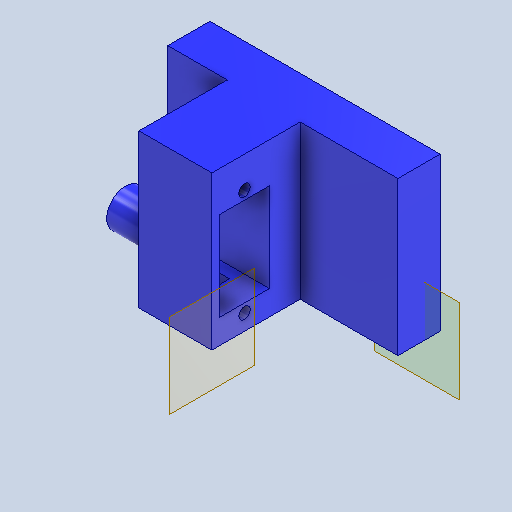
# Autodesk Inventor part: joint5_cover
Saved by Autodesk Inventor 2022 (Build 260153000, 153)
## iProperties
Created: 2024-10-12
Part Number: joint5_cover
Material: 一般
Document SubType Name: Modeling
Designer: acbaf
Density: 1 g/cm^3
Appearance: 青 - 壁塗料 - 光沢
Author: acbaf
Autodesk Inventor part; units mm, degrees
ref_plane "YZ Plane" through (0, 0, 0) normal (1, 0, 0) x (0, 1, 0)
sketch "スケッチ12" plane through (0, 0, 0) normal (1, 0, 0) x (0, 1, 0)
  line L0 (0, 0) -> (-40, 0)
  line L1 (-40, 0) -> (-40, -30)
  line L2 (-40, -30) -> (0, -30)
  line L3 (0, -30) -> (0, 0)
  dimension "d86" = 40
  dimension "d87" = 30
  constraints: 8 end point, 2 parallel, 1 horizontal, 1 perpendicular
  measures "d86" distance of L2.end L1.end
  measures "d87" distance of L1.end L0.end
extrude "押し出し15" add sketch "スケッチ12" along normal blind 60
sketch "スケッチ13" plane through (60, 0, 0) normal (1, 0, 0) x (0, 0, -1)
  line L0 (0, 0) -> (0, -2)
  line L1 (2, -10.4) -> (15, -10.4)
  line L2 (15, -10.4) -> (15, -33.6)
  line L3 (15, -33.6) -> (2, -33.6)
  line L4 (2, -33.6) -> (2, -10.4)
  line L5 (30, 0) -> (0, 0) projected
  line L6 (30, -40) -> (30, 0) projected
  line L7 (0, 0) -> (0, -40) projected
  line L8 (0, -40) -> (30, -40) projected
  line L9 (30, -40) -> (30, 0) projected
  line L10 (30, 0) -> (0, 0) projected
  line L11 (0, 0) -> (0, -40) projected
  line L12 (0, -40) -> (30, -40) projected
  line L13 (23, -40) -> (23, 0)
  point P0 (-10, 3.6606)
  point P1 (23, 0)
  point P2 (8.5, -27.6)
  dimension "d94" = 23.2
  dimension "d95" = 10.4
  dimension "d99" = 13
  dimension "d130" = 8
  dimension "d137" = 6
  dimension "d138" = 6.5
  dimension "d145" = 15
  dimension "d146" = 2
  constraints: 12 end point, 2 parallel, 2 perpendicular, 2 point on line, 1 horizontal
  measures "d94" distance of L1.end L2.end
  measures "d95" distance between parallel lines of L1 L5
  measures "d99" distance of L1.start L1.end
  measures "d130" distance between parallel lines of L13 L2
  measures "d137" distance from line of L3 point (8.5, -27.6)
  measures "d138" distance from line of point (8.5, -27.6) L4
  measures "d145" distance between parallel lines of L2 L6
  measures "d146" distance between parallel lines of L7 L4
extrude "押し出し16" cut sketch "スケッチ13" against normal blind 16.4 contours L1 L2 L3 L4
sketch "スケッチ14" plane through (0, -40, -30) normal (0, 0, -1) x (-1, 0, 0)
  line L0 (0, 0) -> (0, 40) projected
  line L1 (0, 40) -> (-60, 40) projected
  line L2 (-60, 0) -> (-60, 40) projected
  line L3 (0, 0) -> (-60, 0) projected
  circle A0 centre (-30, 20) radius 2.7
  circle A1 centre (-30, 20) radius 4.75
  line L4 (-30, 20) -> (-54, 20)
  line L5 (-30, 20) -> (-6, 20)
  circle A2 centre (-30, 20) radius 6.5
  circle A3 centre (-6, 20) radius 4
  line L6 (-30, 13.5) -> (-30, 26.5)
  circle A4 centre (-54, 20) radius 4
  line L7 (-29.3229, 13.5354) -> (-5.5833, 16.0218)
  line L8 (-5.5833, 23.9782) -> (-29.3229, 26.4646)
  line L9 (-30.6771, 26.4646) -> (-54.4167, 23.9782)
  line L10 (-30.6771, 13.5354) -> (-54.4167, 16.0218)
  circle A5 centre (-54, 20) radius 0.5
  circle A6 centre (-50, 20) radius 0.5
  circle A7 centre (-46, 20) radius 0.5
  circle A8 centre (-42, 20) radius 0.5
  circle A9 centre (-38, 20) radius 0.5
  circle A10 centre (-6, 20) radius 0.5
  circle A11 centre (-10, 20) radius 0.5
  circle A12 centre (-14, 20) radius 0.5
  circle A13 centre (-18, 20) radius 0.5
  circle A14 centre (-22, 20) radius 0.5
  line L11 (44.5, 22.6) -> (44.5, 22.6)
  line L12 (-15.5, 0) -> (-15.5, 0)
  line L13 (-46.2012, 14.0596) -> (-13.7988, 25.9404)
  line L14 (44.5, 0) -> (44.5, 0)
  line L15 (-15.5, 22.6) -> (-15.5, 22.6)
  line L16 (44.5, 22.6) -> (44.5, 22.6)
  line L17 (44.5, 22.6) -> (-15.5, 0)
  line L18 (44.5, 22.6) -> (-15.5, 22.6)
  line L19 (-15.5, 22.6) -> (44.5, 0)
  point P0 (16, 11.6)
  point P1 (-30, 20)
  point P2 (14.5, 11.3)
  dimension "d170" = 5.4
  dimension "d171" = 9.5
  dimension "d172" = 24
  dimension "d173" = 24
  dimension "d174" = 13
  dimension "d175" = 8
  dimension "d176" = 0
  dimension "d177" = 0
  dimension "d178" = 1
  dimension "d179" = 1
  dimension "d180" = 4
  dimension "d181" = 1
  dimension "d182" = 1
  dimension "d183" = 1
  dimension "d184" = 4
  dimension "d185" = 4
  dimension "d186" = 4
  dimension "d187" = 30
  dimension "d188" = 20
  constraints: 32 end point, 15 centre point, 10 point on circle, 8 tangent, 6 coincident, 6 symmetric about line, 5 midpoint, 3 point on line, 6 other
  measures "d170" diameter of A0
  measures "d171" diameter of A1
  measures "d172" distance of L4.start L4.end
  measures "d173" distance of L4.start L5.end
  measures "d174" diameter of A2
  measures "d175" diameter of A3
  measures "d176" distance from line of L4 A4.centre
  measures "d177" distance from line of L6 A0.centre
  measures "d178" diameter of A5
  measures "d179" diameter of A6
  measures "d180" distance of L4.end A6.centre
  measures "d181" diameter of A7
  measures "d182" diameter of A8
  measures "d183" diameter of A9
  measures "d184" distance of A6.centre A7.centre
  measures "d185" distance of A7.centre A8.centre
  measures "d186" distance of A9.centre A8.centre
  measures "d187" distance from line of L2 point (-30, 20)
  measures "d188" distance from line of point (-30, 20) L1
extrude "押し出し17" cut sketch "スケッチ14" against normal blind 4 contours A10 | L19 A11 A3 L18 | A3 A11 L5 L19 | L18 A3 | L7 A2 L5 A14 A13 A12 A11 A3 | L5 A11 L19 | A3 L18 L19 A11 L5 A12 A13 A14 A2 L13 L8 | A3 L19 L18 | A11 L5 A3 | A3 L5 A11 | A2 L6 A1 L5 | L5 A3 A11 L19 | L19 A11 | L13 A2 L8 | L19 A11 A3 | L5 A11 A3 | A2 L13 A1 L6 | L5 A1 L13 A2 | A2 L13 A1 L6 | A12 L5 | L5 A12 | L10 L13 A2 | L6 A0 L5 A1 | A1 L13 A0 L6 | L5 A0 L13 A1 | A14 L5 | L5 A14 | L6 A1 L4 A2 | L13 A0 L6 A1 | L13 L10 A4 A6 L4 A7 A8 A9 A2 | A2 L4 A1 L13 | A1 L4 A0 L13 | L6 L5 A0 | A0 L13 L6 | L5 L13 A0 | A2 L4 A9 A8 A7 A6 A4 L9 | L6 A0 L4 A1 | L13 L6 A0 | A13 L5 | L5 A13 | A5 | A4 A6 | A0 L4 L13 | L4 A0 L6 | A9 L4 | L4 A9 | A6 L4 A4 | A4 L4 A6 | A6 L4 A4 | A4 L4 A6 | A8 L4 | L4 A8 | A7 L4 | L4 A7
ref_plane "作業平面3" through (25, 0, 0) normal (1, 0, 0) x (0, 0, -1)
ref_plane "作業平面4" through (34.5, 0, 0) normal (1, 0, 0) x (0, 0, -1)
ref_plane "作業平面5" through (15.5, 0, 0) normal (1, 0, 0) x (0, 0, -1)
sketch "スケッチ15" plane through (34.5, 0, 0) normal (1, 0, 0) x (0, 0, -1)
  line L0 (2, -10.4) -> (15, -10.4) projected
  line L1 (15, -33.6) -> (2, -33.6) projected
  line L2 (15, -10.4) -> (15, -33.6) projected
  line L3 (2, -10.4) -> (15, -10.4) projected
  line L4 (2, -33.6) -> (2, -10.4) projected
  point P0 (0, 0)
extrude "押し出し19" cut sketch "スケッチ13" along normal blind 30 from surface at -25.5 contours L5 L13 L8 L7 L0 | L1 L2 L3 L4
extrude "押し出し20" cut sketch "スケッチ13" against normal blind 30 from surface at -44.5 contours L5 L13 L8 L7 L0 | L1 L2 L3 L4
extrude "押し出し21" cut sketch "スケッチ13" against normal blind 16.4 from surface at -25.5 contours L1 L2 L3 L4
sketch "スケッチ16" plane through (15.5, 0, 0) normal (1, 0, 0) x (0, 0, -1)
  line L0 (23, 0) -> (23, -40) projected
  line L1 (0, -40) -> (23, -40) projected
  line L2 (0, 0) -> (0, -40) projected
  line L3 (23, 0) -> (0, 0) projected
  line L4 (15, -33.6) -> (2, -33.6) projected
  line L5 (2, -33.6) -> (2, -10.4) projected
  line L6 (15, -10.4) -> (15, -33.6) projected
  line L7 (2, -10.4) -> (15, -10.4) projected
  circle A0 centre (8.5, -27.6) radius 4.9
  dimension "d140" = 6
  dimension "d141" = 6.5
  dimension "d142" = 9.8
  constraints: 1 centre point, 1 coincident
  measures "d140" distance from line of L4 point (8.5, -27.6)
  measures "d141" distance from line of L5 point (8.5, -27.6)
  measures "d142" diameter of A0
extrude "押し出し22" add sketch "スケッチ16" against normal blind 12 contours A0
sketch "スケッチ17" plane through (18.1, -33.6, -2) normal (0, 1, 0) x (1, 0, 0)
  line L0 (2, 10) -> (9, 10)
  line L1 (9, 10) -> (9, 3)
  line L2 (9, 3) -> (2, 3)
  line L3 (2, 3) -> (2, 10)
  line L4 (0, 13) -> (0, 0) projected
  line L5 (0, 13) -> (16.4, 13) projected
  point P0 (-18.1, -2)
  dimension "d147" = 7
  dimension "d148" = 7
  dimension "d149" = 2
  dimension "d150" = 3
  constraints: 8 end point, 2 parallel, 1 horizontal, 1 perpendicular
  measures "d147" distance of L1.end L2.end
  measures "d148" distance of L0.end L1.end
  measures "d149" distance between parallel lines of L3 L4
  measures "d150" distance between parallel lines of L5 L0
extrude "押し出し23" cut sketch "スケッチ17" against normal blind 10
extrude "押し出し24" cut sketch "スケッチ14" against normal blind 1.5 from surface at -4 contours L6 L5 A0 | A0 L13 L6 | L5 L13 A0 | L13 L6 A0 | A0 L4 L13 | L4 A0 L6
ref_plane "作業平面7" through (58, -38, -30) normal (0, 0, -1) x (-1, 0, 0)
sketch "スケッチ18" plane through (58, -38, -30) normal (0, 0, -1) x (-1, 0, 0)
  circle A0 centre (27.1663, 23.0232) radius 2.7 projected
  line L0 (51.583, 19.0449) -> (27.8434, 16.5585) projected
  arc A1 (51.583, 19.0449) -> (51.583, 27.0014) centre (51.1663, 23.0232) ccw projected
  line L1 (27.8434, 29.4878) -> (51.583, 27.0014) projected
  arc A2 (27.8434, 29.4878) -> (26.4892, 29.4878) centre (27.1663, 23.0232) ccw projected
  line L2 (2.7497, 27.0014) -> (26.4892, 29.4878) projected
  arc A3 (2.7497, 27.0014) -> (2.7497, 19.0449) centre (3.1663, 23.0232) ccw projected
  line L3 (26.4892, 16.5585) -> (2.7497, 19.0449) projected
  arc A4 (26.4892, 16.5585) -> (27.8434, 16.5585) centre (27.1663, 23.0232) ccw projected
  line L4 (3.5833, 21.9782) -> (27.3229, 24.4646) projected
  line L5 (52.4167, 14.0218) -> (28.6771, 11.5354) projected
  arc A5 (52.4167, 14.0218) -> (52.4167, 21.9782) centre (52, 18) ccw projected
  line L6 (28.6771, 24.4646) -> (52.4167, 21.9782) projected
  arc A6 (28.6771, 24.4646) -> (27.3229, 24.4646) centre (28, 18) ccw projected
  line L7 (3.5833, 21.9782) -> (27.3229, 24.4646) projected
  arc A7 (3.5833, 21.9782) -> (3.5833, 14.0218) centre (4, 18) ccw projected
  line L8 (27.3229, 11.5354) -> (3.5833, 14.0218) projected
  arc A8 (27.3229, 11.5354) -> (28.6771, 11.5354) centre (28, 18) ccw projected
  arc A9 (3.5521, 22.2766) -> (3.5521, 13.7234) centre (4, 18) ccw
  line L9 (3.5521, 22.2766) -> (27.2917, 24.763)
  arc A10 (28.7083, 24.763) -> (27.2917, 24.763) centre (28, 18) ccw
  line L10 (28.7083, 24.763) -> (52.4479, 22.2766)
  arc A11 (52.4479, 13.7234) -> (52.4479, 22.2766) centre (52, 18) ccw
  line L11 (52.4479, 13.7234) -> (28.7083, 11.237)
  arc A12 (27.2917, 11.237) -> (28.7083, 11.237) centre (28, 18) ccw
  line L12 (27.2917, 11.237) -> (3.5521, 13.7234)
  point P0 (58, 38)
  dimension "d189" = 0.3
  constraints: 8 end point, 8 point on circle, 4 centre point, 7 other
  measures "d189" distance between parallel lines of L8 L12
extrude "押し出し25" cut sketch "スケッチ18" against normal blind 4 contours L6 A6 L4 A0 L9 A10 L10 | A0 L10 A11 A1 A5 L6 | L4 A7 A3 A9 L9 A0 | A1 A11 L11 A12 L12 A9 A3 A7 L8 A8 L5 A5
extrude "押し出し26" cut sketch "スケッチ14" against normal blind 2 from surface at -4 contours A11 L5 A3 | A3 L5 A11 | L5 A3 A11 L19 | L19 A11 | L5 A11 A3 | A6 L4 A4 | A4 L4 A6 | A6 L4 A4 | A4 L4 A6 picked at (-9.8359, 20.0907)
ref_plane "作業平面6" through (34.5, -38, 0) normal (1, 0, 0) x (0, 0, -1)
sketch "スケッチ19" plane through (34.5, -38, 0) normal (1, 0, 0) x (0, 0, -1)
  line L0 (2, 4.4) -> (2, 27.6) projected
  line L1 (2, 27.6) -> (15, 27.6) projected
  line L2 (15, 27.6) -> (15, 4.4) projected
  line L3 (15, 4.4) -> (2, 4.4) projected
  circle A0 centre (8.5, 2.15) radius 1.5
  circle A1 centre (8.5, 29.85) radius 1.5
  point P0 (0, 38)
  dimension "d161" = 3
  dimension "d162" = 3
  dimension "d163" = 2.25
  dimension "d164" = 2.25
  dimension "d165" = 6.5
  dimension "d167" = 6.5
  constraints: 2 centre point
  measures "d161" diameter of A0
  measures "d162" diameter of A1
  measures "d163" distance from line of L1 A1.centre
  measures "d164" distance from line of L3 A0.centre
  measures "d165" distance from line of A1.centre L0
  measures "d167" distance from line of L0 A0.centre
extrude "押し出し27" cut sketch "スケッチ19" against normal blind 4 contours A0 | A1
sketch "スケッチ20" plane through (0, -40, -30) normal (0, 0, -1) x (-1, 0, 0)
  arc A0 (-29.2917, 26.763) -> (-30.7083, 26.763) centre (-30, 20) ccw projected
  line L0 (-29.2917, 26.763) -> (-5.5521, 24.2766) projected
  arc A1 (-5.5521, 15.7234) -> (-5.5521, 24.2766) centre (-6, 20) ccw projected
  line L1 (-5.5521, 15.7234) -> (-29.2917, 13.237) projected
  arc A2 (-30.7083, 13.237) -> (-29.2917, 13.237) centre (-30, 20) ccw projected
  line L2 (-30.7083, 13.237) -> (-54.4479, 15.7234) projected
  arc A3 (-54.4479, 24.2766) -> (-54.4479, 15.7234) centre (-54, 20) ccw projected
  line L3 (-54.4479, 24.2766) -> (-30.7083, 26.763) projected
  line L4 (0, 40) -> (-60, 40) projected
  line L5 (-60, 0) -> (-60, 40) projected
  line L6 (0, 0) -> (-60, 0) projected
  line L7 (0, 0) -> (0, 40) projected
  point P0 (0, 40)
extrude "押し出し28" add sketch "スケッチ20" along normal blind 4
